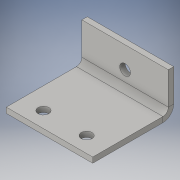
# Autodesk Inventor part: Sheet for
Saved by Autodesk Inventor 2016 SP2 (Build 200236200, 236)
## iProperties
Created: 2018-01-31
Part Number: Sheet for
Material: Generic
Document SubType Name: Sheet Metal
Designer: CAD
Density: 1 g/cm^3
Sheet Metal Rule: Default
Appearance: Default
Author: CAD
Autodesk Inventor part; units mm, degrees
ref_plane "YZ Plane" through (0, 0, 0) normal (1, 0, 0) x (0, 1, 0)
ref_plane "XZ Plane" through (0, 0, 0) normal (0, 1, 0) x (-1, 0, 0)
ref_plane "XY Plane" through (0, 0, 0) normal (0, 0, 1) x (1, 0, 0)
sketch "Sketch1" plane through (0, 0, 0) normal (0, 1, 0) x (-1, 0, 0)
  line L0 (25.4, 25.4) -> (-25.4, 25.4)
  line L1 (-25.4, 25.4) -> (-25.4, -22.225)
  line L2 (-25.4, -22.225) -> (25.4, -22.225)
  line L3 (25.4, -22.225) -> (25.4, 25.4)
  point P0 (0, 0)
  dimension "d0" = 50.8
  dimension "d1" = 47.625
  dimension "d2" = 25.4
  dimension "d3" = 25.4
  constraints: 8 end point, 2 parallel, 1 horizontal, 1 perpendicular
  measures "d0" distance of L2.end L1.end
  measures "d1" distance of L1.end L0.end
  measures "d2" distance from line of point (0, 0) L3
  measures "d3" distance from line of L0 point (0, 0)
extrude "Extrusion1" add sketch "Sketch1" along normal blind 3.175
sketch "Sketch4" plane through (-25.4, 0, -19.05) normal (0, 0, -1) x (-1, 0, 0)
  line L0 (-50.8, 0) -> (0, 0)
  line L1 (0, 0) -> (0, 25.4)
  line L2 (0, 25.4) -> (-50.8, 25.4)
  line L3 (-50.8, 25.4) -> (-50.8, 0)
  constraints: 6 end point, 1 horizontal, 1 perpendicular, 1 vertical
edge flange "Flange1" height 25.4 angle 90 thickness 3.175 bend radius 3.175 thickness toward (0, 0, -1) relief straight relief width 3.175 relief depth 1.5875 edges at (0, 3.175, -22.225) wall of the first edge with corners at (25.4, 0, -19.05) (-25.4, 0, -19.05) (-25.4, 25.4, -19.05) (25.4, 25.4, -19.05)
bend "Bend1"
corner "Corner1"
sketch "Sketch5" plane through (0, 3.175, 0) normal (0, 1, 0) x (1, 0, 0)
  line L0 (-25.4, -25.4) -> (25.4, -25.4) projected
  line L1 (-25.4, 15.875) -> (-25.4, -25.4) projected
  point P0 (0, 0)
  point P1 (-12.7, -16.256)
  point P2 (12.7, -16.256)
  dimension "d23" = 9.144
  dimension "d24" = 9.144
  dimension "d25" = 25.4
  dimension "d26" = 12.7
  measures "d23" distance from line of L0 point (12.7, -16.256)
  measures "d24" distance from line of L0 point (-12.7, -16.256)
  measures "d25" distance of point (12.7, -16.256) point (-12.7, -16.256)
  measures "d26" distance from line of L1 point (-12.7, -16.256)
hole "Hole1" at (-12.7, 3.175, 16.256) at (12.7, 3.175, 16.256) direction (0, -1, 0) diameter 6.35 end through all
sketch "Sketch6" plane through (25.4, 25.4, -22.225) normal (0, 0, -1) x (-1, 0, 0)
  line L0 (0, 0) -> (50.8, 0) projected
  line L1 (50.8, 0) -> (50.8, -19.05) projected
  point P0 (25.4, -25.4)
  point P1 (25.4, -12.7)
  dimension "d34" = 12.7
  dimension "d35" = 25.4
  measures "d34" distance from line of L0 point (25.4, -12.7)
  measures "d35" distance from line of point (25.4, -12.7) L1
hole "Hole2" at (0, 12.7, -22.225) direction (0, 0, 1) diameter 6.35 end through all
equation "\"d24\" = d23"
equation "\"d32\" = Thickness"
equation "\"d41\" = Thickness"
equation "\"d13\" = BendReliefWidth"
equation "\"d14\" = BendReliefDepth"
equation "\"d15\" = MinimumRemnant"
equation "\"d16\" = BendRadius"
equation "\"d19\" = BendRadius"
equation "\"d20\" = CornerReliefSize"
equation "\"d21\" = GapSize"
equation "\"d22\" = JacobiRadiusSize"
equation "\"BendRadius\" = Thickness"
equation "\"BendReliefWidth\" = Thickness"
equation "\"BendReliefDepth\" = 0.5 * Thickness"
equation "\"CornerReliefSize\" = 4 * Thickness"
equation "\"MinimumRemnant\" = 2 * Thickness"
equation "\"TransitionRadius\" = BendRadius"
equation "\"JacobiRadiusSize\" = BendRadius"
equation "\"GapSize\" = Thickness"
equation "\"Thickness\" = 3.175"
body "Solid1"
